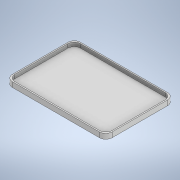
# Autodesk Inventor part: víko
Saved by Autodesk Inventor 2021 (Build 250183000, 183)
## iProperties
Created: 2020-12-03
Part Number: víko
Material: Všeobecné
Document SubType Name: Modeling
Designer: Adam
Density: 1 g/cm^3
Appearance: Výchozí
Author: Adam
Autodesk Inventor part; units mm, degrees
ref_plane "YZ Plane" through (0, 0, 0) normal (1, 0, 0) x (0, 1, 0)
ref_plane "XZ Plane" through (0, 0, 0) normal (0, 1, 0) x (-1, 0, 0)
ref_plane "XY Plane" through (0, 0, 0) normal (0, 0, 1) x (1, 0, 0)
sketch "Náčrt1" plane through (0, 0, 0) normal (0, 1, 0) x (-1, 0, 0)
  line L0 (0, 0) -> (-158, 0)
  line L1 (-158, 0) -> (-158, -108)
  line L2 (-158, -108) -> (0, -108)
  line L3 (0, -108) -> (0, 0)
  dimension "d0" = 158
  dimension "d1" = 108
  constraints: 8 end point, 2 parallel, 1 horizontal, 1 perpendicular
  measures "d0" distance of L2.end L1.end
  measures "d1" distance of L1.end L0.end
extrude "Vysunutí1" add sketch "Náčrt1" along normal blind 8
sketch "Náčrt2" plane through (0, 8, 0) normal (0, 1, 0) x (1, 0, 0)
  line L0 (2, 2) -> (156, 2)
  line L1 (156, 2) -> (156, 106)
  line L2 (156, 106) -> (2, 106)
  line L3 (2, 106) -> (2, 2)
  line L4 (0, 108) -> (0, 0) projected
  line L5 (0, 0) -> (158, 0) projected
  dimension "d4" = 154
  dimension "d5" = 104
  dimension "d6" = 2
  dimension "d7" = 2
  constraints: 8 end point, 2 parallel, 1 horizontal, 1 perpendicular
  measures "d4" distance of L2.end L1.end
  measures "d5" distance of L1.end L0.end
  measures "d6" distance between parallel lines of L4 L3
  measures "d7" distance between parallel lines of L5 L0
extrude "Vysunutí2" cut sketch "Náčrt2" against normal blind 6
fillet "Zaoblení1" radius 10 8 edges at (156, 5, -106) (158, 4, -108) (158, 4, 0) (0, 4, 0) (2, 5, -106) (0, 4, -108) (156, 5, -2) (2, 5, -2)
